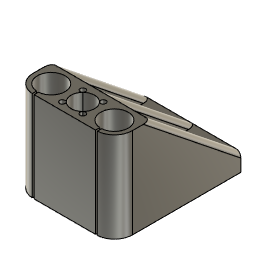
Z-Carriage (Autodesk Fusion 360 design; units mm, degrees)
Autodesk Fusion 360 part; units mm, degrees
sketch "Skizze1" plane through (0, 0, 0) normal (0, 0, 1) x (1, 0, 0)
  line L0 (0, 0) -> (55, 0)
  line L1 (55, 0) -> (55, 70)
  line L2 (55, 70) -> (0, 70)
  line L3 (0, 70) -> (0, 0)
  line L4 (0, 10) -> (55, 10)
  circle A0 centre (10, 10) radius 7.65
  circle A1 centre (45, 10) radius 7.65
  line L5 (27.5, 0) -> (27.5, 10)
  line L6 (0, 20) -> (55, 20)
  line L7 (9.5, 5) -> (10.5, 5)
  line L8 (10.5, 5) -> (10.5, 0)
  line L9 (10.5, 0) -> (9.5, 0)
  line L10 (9.5, 0) -> (9.5, 5)
  line L11 (44.5, 0) -> (45.5, 0)
  line L12 (45.5, 0) -> (45.5, 5)
  line L13 (45.5, 5) -> (44.5, 5)
  line L14 (44.5, 5) -> (44.5, 0)
  circle A2 centre (27.5, 10) radius 8
  line L15 (27.5, 10) -> (33.1569, 15.6569)
  line L16 (27.5, 10) -> (36.1335, 10) construction
  line L17 (27.5, 10) -> (21.8431, 15.6569)
  line L18 (27.5, 10) -> (37.9731, 10) construction
  line L19 (27.5, 10) -> (33.1569, 4.3431)
  line L20 (27.5, 10) -> (37.3995, 10) construction
  line L21 (27.5, 10) -> (21.8431, 4.3431)
  line L22 (27.5, 10) -> (35.5, 10) construction
  circle A3 centre (21.8431, 15.6569) radius 1.5
  circle A4 centre (33.1569, 15.6569) radius 1.5
  circle A5 centre (33.1569, 4.3431) radius 1.5
  circle A6 centre (21.8431, 4.3431) radius 1.5
  line L23 (0, 70) -> (5, 70)
  line L24 (5, 70) -> (5, 20)
  line L25 (5, 20) -> (0, 20)
  line L26 (0, 20) -> (0, 70)
  line L27 (55, 70) -> (50, 70)
  line L28 (50, 70) -> (50, 20)
  line L29 (50, 20) -> (55, 20)
  line L30 (55, 20) -> (55, 70)
  line L31 (30, 70) -> (25, 70)
  line L32 (25, 70) -> (25, 20)
  line L33 (25, 20) -> (30, 20)
  line L34 (30, 20) -> (30, 70)
  circle A7 centre (27.5, 10) radius 6.5
  circle A8 centre (27.5, 10) radius 7.25
  line L35 (5, 60) -> (50, 60)
  dimension "d1" = 55
  dimension "d2" = 70
  dimension "d3" = 10
  dimension "d4" = 15.3
  dimension "d5" = 15.3
  dimension "d6" = 17.5
  dimension "d7" = 17.5
  dimension "d8" = 20
  dimension "d9" = 1
  dimension "d10" = 5
  dimension "d11" = 0.5
  dimension "d12" = 1
  dimension "d13" = 5
  dimension "d14" = 0.5
  dimension "d15" = 16
  dimension "d16" = 45
  dimension "d17" = 135
  dimension "d19" = 45
  dimension "d20" = 135
  dimension "d21" = 3
  dimension "d22" = 3
  dimension "d23" = 3
  dimension "d24" = 3
  dimension "d29" = 5
  dimension "d30" = 50
  dimension "d31" = 5
  dimension "d32" = 50
  dimension "d33" = 5
  dimension "d34" = 50
  dimension "d35" = 25
  dimension "d40" = 13
  dimension "d41" = 14.5
  dimension "d52" = 10
  constraint horizontal L0
  constraint vertical L1
  constraint horizontal L2
  constraint vertical L3
  constraint coincident L0.start L3.end
  constraint coincident L3 L4.start
  constraint coincident L1 L4.end
  constraint perpendicular L1 L4
  constraint coincident L4 A0.centre
  constraint coincident L4 A1.centre
  constraint midpoint L0 L5.start
  constraint midpoint L4 L5.end
  constraint coincident L3 L6.start
  constraint coincident L1 L6.end
  constraint perpendicular L1 L6
  constraint horizontal L7
  constraint vertical L8
  constraint horizontal L9
  constraint vertical L10
  constraint collinear L0 L9
  constraint horizontal L11
  constraint vertical L12
  constraint horizontal L13
  constraint vertical L14
  constraint collinear L0 L11
  constraint coincident L5.end A2.centre
  constraint horizontal L16
  constraint horizontal L18
  constraint horizontal L20
  constraint coincident A2 L17.end
  constraint coincident A2 L15.end
  constraint coincident A2 L19.end
  constraint horizontal L22
  constraint coincident L17.end A3.centre
  constraint coincident L15.end A4.centre
  constraint coincident L19.end A5.centre
  constraint coincident L21.end A6.centre
  constraint horizontal L23
  constraint vertical L24
  constraint horizontal L25
  constraint vertical L26
  constraint horizontal L27
  constraint vertical L28
  constraint horizontal L29
  constraint vertical L30
  constraint horizontal L31
  constraint vertical L32
  constraint horizontal L33
  constraint vertical L34
  constraint coincident L2 L31.start
  constraint coincident L24 L35.start
  constraint coincident L28 L35.end
  constraint perpendicular L28 L35
  measures "d1" distance of L0.start L0.end
  measures "d2" distance of L0.start L2.end
  measures "d3" distance of L0 L4
  measures "d4" diameter of A0
  measures "d5" diameter of A1
  measures "d6" distance of A0.centre L5
  measures "d7" distance of A1.centre L5
  measures "d8" distance of L0 L6
  measures "d9" distance of L7.start L7.end
  measures "d10" distance of L7.start L9.end
  measures "d11" distance of A0.centre L10
  measures "d12" distance of L11.start L11.end
  measures "d13" distance of L11.start L13.end
  measures "d14" distance of A1.centre L14
  measures "d15" diameter of A2
  measures "d16" angle of L15 L16
  measures "d17" angle of L17 L18
  measures "d19" angle of L19 L20
  measures "d20" angle of L21 L22
  measures "d21" diameter of A3
  measures "d22" diameter of A4
  measures "d23" diameter of A5
  measures "d24" diameter of A6
  measures "d29" distance of L2.end L23.end
  measures "d30" distance of L2.end L6.start
  measures "d31" distance of L1.end L27.end
  measures "d32" distance of L1.end L6.end
  measures "d33" distance of L31.start L31.end
  measures "d34" distance of L31.start L33.end
  measures "d35" distance of L3 L32
  measures "d40" diameter of A7
  measures "d41" diameter of A8
  measures "d52" distance of L2 L35
extrude "Extrusion1" add sketch "Skizze1" along normal blind 50 contours L0 L3 L4 A0 L10 | L1 L3 L4 A0 A1 L6 A2 A3 A4 L25 L29 L33 | L0 L4 A0 L5 L8 A2 A6 | L2 L3 L6 L23 L24 L25 L26 | L0 L4 A1 L5 L14 A2 A5 | L5 A2 A6 A8 | L5 A2 A5 A8 | L6 L32 L33 L34 L35 | L4 A2 A3 A8 | L4 A2 A6 A8 | L0 L1 L4 A1 L12 | L5 A6 A7 A8 | L5 A5 A7 A8 | L2 L31 L32 L34 L35 | L4 A3 A7 A8 | L4 A6 A7 A8 | L1 L2 L6 L27 L28 L29 L30 | A2 A3 A4 A8 | L4 A2 A5 A8 | L4 A2 A4 A8 | L4 A5 A7 A8 | A3 A4 A7 A8 | L4 A4 A7 A8
extrude "Extrusion2" add sketch "Skizze1" along normal blind 10 contours L2 L3 L6 L23 L24 L25 L26 | L2 L24 L32 L35 | L6 L32 L33 L34 L35 | L2 L31 L32 L34 L35 | L2 L28 L34 L35 | L1 L2 L6 L27 L28 L29 L30
sketch "Skizze2" plane through (55, 0, 0) normal (1, 0, 0) x (0, 1, 0)
  line L0 (70, 0) -> (70, 50)
  line L1 (70, 50) -> (0, 50)
  line L2 (0, 50) -> (0, 0)
  line L3 (0, 0) -> (70, 0)
  line L4 (0, 50) -> (20, 50)
  line L5 (70, 0) -> (70, 10)
  line L6 (20, 50) -> (70, 10)
  line L7 (70, 10) -> (70, 50)
  line L8 (70, 50) -> (20, 50)
  dimension "d36" = 10
  dimension "d37" = 20
  constraint coincident L1.end L2.start
  constraint coincident L1 L4.end
  constraint perpendicular L2 L4
  constraint coincident L0.start L3.end
  constraint perpendicular L3 L5
  constraint coincident L0.end L1.start
  measures "d36" distance of L0.start L5.end
  measures "d37" distance of L1.end L4.end
extrude "Extrusion3" cut sketch "Skizze2" against normal blind 55 contours L0 L1 L6 L7 L8
extrude "Extrusion4" cut sketch "Skizze1" along normal blind 37 contours L5 A6 A7 A8 | L5 A5 A7 A8 | L4 A3 A7 A8 | L4 A6 A7 A8 | L4 A5 A7 A8 | A3 A4 A7 A8 | L4 A4 A7 A8
chamfer "Fase1" distance 0.75 angle 45 4 edges at (34.75, 10, 37) (27.5, 17.25, 37) (20.25, 10, 37) (27.5, 2.75, 37)
sketch "Skizze3" plane through (0, 70, 0) normal (0, 1, 0) x (-1, 0, 0)
  line L0 (-50, 10) -> (-55, 10)
  line L1 (-55, 10) -> (-55, 0)
  line L2 (-55, 0) -> (0, 0)
  line L3 (0, 0) -> (0, 10)
  line L4 (0, 10) -> (-5, 10)
  line L5 (-5, 10) -> (-25, 10)
  line L6 (-25, 10) -> (-30, 10)
  line L7 (-30, 10) -> (-50, 10)
  line L8 (-55, 5) -> (0, 5)
  line L9 (-27.5, 0) -> (-27.5, 10)
  circle A0 centre (-27.5, 5) radius 1.5
  circle A1 centre (-37.5, 5) radius 1.5
  circle A2 centre (-47.5, 5) radius 1.5
  circle A3 centre (-17.5, 5) radius 1.5
  circle A4 centre (-7.5, 5) radius 1.5
  dimension "d45" = 3
  dimension "d46" = 10
  dimension "d47" = 10
  dimension "d48" = 10
  dimension "d49" = 10
  constraint midpoint L1 L8.start
  constraint midpoint L3 L8.end
  constraint midpoint L2 L9.start
  constraint midpoint L6 L9.end
  constraint midpoint L8 A0.centre
  constraint coincident L8 A1.centre
  constraint coincident L8 A2.centre
  constraint coincident L8 A3.centre
  constraint coincident L8 A4.centre
  constraint equal A1 A2
  constraint equal A0 A1
  constraint equal A0 A3
  constraint equal A3 A4
  measures "d45" diameter of A0
  measures "d46" distance of A0.centre A1.centre
  measures "d47" distance of A1.centre A2.centre
  measures "d48" distance of A0.centre A3.centre
  measures "d49" distance of A3.centre A4.centre
extrude "Extrusion5" cut sketch "Skizze3" against normal blind 15 contours L8 A2 | L8 A2 | L8 L9 A0 | L8 L9 A0 | L8 L9 A0 | L8 L9 A0 | L8 A1 | L8 A1 | L8 A3 | L8 A3 | L8 A4 | L8 A4
fillet "Abrundung1" radius 10 2 edges at (55, 0, 25) (0, 0, 25)
fillet "Abrundung2" radius 2.5 6 edges at (30, 45, 30) (25, 45, 30) (0, 45, 30) (5, 45, 30) (50, 45, 30) (55, 45, 30)
